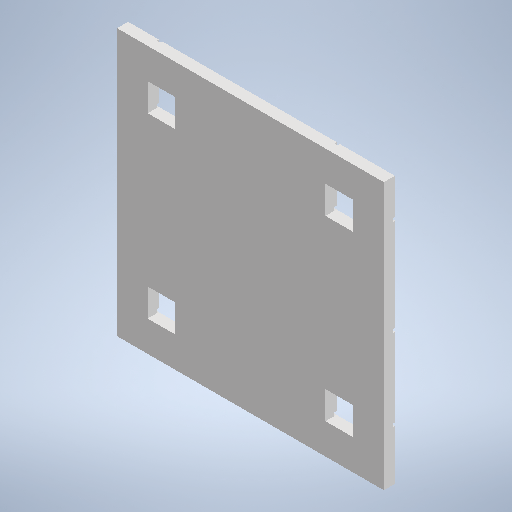
# Autodesk Inventor part: LED Position
Saved by Autodesk Inventor 2025.2 (Build 292293000, 293)
## iProperties
Created: 2025-04-29
Part Number: LED Position
Material: Generic
Document SubType Name: Modeling
Designer: powel
Density: 1 g/cm^3
Appearance: Default
Author: powel
Autodesk Inventor part; units mm, degrees
ref_plane "YZ Plane" through (0, 0, 0) normal (1, 0, 0) x (0, 1, 0)
ref_plane "XZ Plane" through (0, 0, 0) normal (0, 1, 0) x (-1, 0, 0)
ref_plane "XY Plane" through (0, 0, 0) normal (0, 0, 1) x (1, 0, 0)
sketch "Sketch1" plane through (0, 0, 0) normal (0, 0, 1) x (1, 0, 0)
  line L0 (0, 0) -> (48, 0)
  line L1 (48, 0) -> (48, 48)
  line L2 (48, 48) -> (0, 48)
  line L3 (0, 48) -> (0, 0)
  line L4 (10.5, 10.5) -> (5.5, 10.5)
  line L5 (5.5, 10.5) -> (5.5, 5.5)
  line L6 (5.5, 5.5) -> (10.5, 5.5)
  line L7 (10.5, 5.5) -> (10.5, 10.5)
  line L8 (10.5, 10.5) -> (5.5, 5.5) construction
  line L9 (5.5, 10.5) -> (10.5, 5.5) construction
  line L10 (5.5, 42.5) -> (10.5, 42.5)
  line L11 (10.5, 42.5) -> (10.5, 37.5)
  line L12 (10.5, 37.5) -> (5.5, 37.5)
  line L13 (5.5, 37.5) -> (5.5, 42.5)
  line L14 (5.5, 42.5) -> (10.5, 37.5) construction
  line L15 (10.5, 42.5) -> (5.5, 37.5) construction
  line L16 (42.5, 5.5) -> (37.5, 5.5)
  line L17 (37.5, 5.5) -> (37.5, 10.5)
  line L18 (37.5, 10.5) -> (42.5, 10.5)
  line L19 (42.5, 10.5) -> (42.5, 5.5)
  line L20 (42.5, 5.5) -> (37.5, 10.5) construction
  line L21 (37.5, 5.5) -> (42.5, 10.5) construction
  line L22 (42.5, 42.5) -> (37.5, 42.5)
  line L23 (37.5, 42.5) -> (37.5, 37.5)
  line L24 (37.5, 37.5) -> (42.5, 37.5)
  line L25 (42.5, 37.5) -> (42.5, 42.5)
  line L26 (42.5, 42.5) -> (37.5, 37.5) construction
  line L27 (37.5, 42.5) -> (42.5, 37.5) construction
  line L28 (37.5, 5.5) -> (37.5, 6.1)
  line L29 (37.5, 6.1) -> (10.5, 10.5)
  line L30 (37.5, 5.5) -> (10.5, 9.9)
  line L31 (37.5, 37.5) -> (37.5, 38.1)
  line L32 (37.5, 38.1) -> (10.5, 42.5)
  line L33 (37.5, 37.5) -> (10.5, 41.9)
  line L34 (0, 24) -> (0, 23.7)
  line L35 (0, 23.7) -> (48, 23.7)
  line L36 (48, 23.7) -> (48, 24.3)
  line L37 (48, 24.3) -> (0, 24.3)
  line L38 (0, 24.3) -> (0, 23.7)
  line L39 (5.5, 10.5) -> (6.1, 10.5)
  line L40 (6.1, 10.5) -> (6.1, 23.7)
  line L41 (6.1, 23.7) -> (5.5, 23.7)
  line L42 (5.5, 23.7) -> (5.5, 10.5)
  line L43 (10.5, 37.5) -> (9.9, 37.5)
  line L44 (9.9, 37.5) -> (9.9, 24.3)
  line L45 (9.9, 24.3) -> (10.5, 24.3)
  line L46 (10.5, 24.3) -> (10.5, 37.5)
  line L47 (37.5, 10.5) -> (38.1, 10.5)
  line L48 (38.1, 10.5) -> (38.1, 23.7)
  line L49 (38.1, 23.7) -> (37.5, 23.7)
  line L50 (37.5, 23.7) -> (37.5, 10.5)
  line L51 (42.5, 37.5) -> (41.9, 37.5)
  line L52 (41.9, 37.5) -> (41.9, 24.3)
  line L53 (41.9, 24.3) -> (42.5, 24.3)
  line L54 (42.5, 24.3) -> (42.5, 37.5)
  line L55 (10.5, 5.5) -> (9.9, 5.5)
  line L56 (9.9, 5.5) -> (9.9, 0)
  line L57 (9.9, 0) -> (10.5, 0)
  line L58 (10.5, 0) -> (10.5, 5.5)
  line L59 (42.5, 5.5) -> (41.9, 5.5)
  line L60 (41.9, 5.5) -> (41.9, 0)
  line L61 (41.9, 0) -> (42.5, 0)
  line L62 (42.5, 0) -> (42.5, 5.5)
  line L63 (37.5, 42.5) -> (38.1, 42.5)
  line L64 (38.1, 42.5) -> (38.1, 48)
  line L65 (38.1, 48) -> (37.5, 48)
  line L66 (37.5, 48) -> (37.5, 42.5)
  line L67 (5.5, 42.5) -> (6.1, 42.5)
  line L68 (6.1, 42.5) -> (6.1, 48)
  line L69 (6.1, 48) -> (5.5, 48)
  line L70 (5.5, 48) -> (5.5, 42.5)
  line L71 (5.5, 37.5) -> (0, 38.4621)
  line L72 (5.5, 37.5) -> (11.0835, 37.5) construction
  line L73 (5.5, 37.5) -> (5.5, 38.1)
  line L74 (5.5, 38.1) -> (0, 38.9963)
  line L75 (5.5, 5.5) -> (0, 6.4621)
  line L76 (5.5, 5.5) -> (11.0835, 5.5) construction
  line L77 (5.5, 5.5) -> (5.5, 6.1)
  line L78 (5.5, 6.1) -> (0, 6.9963)
  line L79 (42.5, 10.5) -> (48, 9.5379)
  line L80 (42.5, 10.5) -> (48.0835, 10.5) construction
  line L81 (42.5, 10.5) -> (42.5, 9.9)
  line L82 (42.5, 9.9) -> (48, 9.0037)
  line L83 (42.5, 42.5) -> (48, 41.6037)
  line L84 (42.5, 42.5) -> (42.5, 41.9)
  line L85 (42.5, 41.9) -> (48, 41.0037)
  line L86 (6.1, 24.3) -> (9.9, 24.3)
  line L87 (10.5, 24.3) -> (12.4, 24.3)
  arc A0 (12.4, 24.3) -> (8, 24.3) centre (10.2, 24.3124) ccw
  line L88 (5.5, 23.7) -> (3.6, 23.7)
  arc A1 (3.6, 23.7) -> (8, 23.7) centre (5.8, 23.7) ccw
  line L89 (41.9, 24.3) -> (40, 24.3)
  line L90 (42.5, 24.3) -> (44.4, 24.3)
  line L91 (37.5, 23.7) -> (35.6, 23.7)
  arc A2 (35.6, 23.7) -> (40, 23.7) centre (37.8, 23.7) ccw
  arc A3 (44.4, 24.3) -> (40, 24.3) centre (42.2, 24.3124) ccw
  point P0 (8, 24.3)
  point P1 (9.9, 26.4919)
  point P2 (41.9, 26.4919)
  point P3 (10.5, 26.4919)
  point P4 (42.5, 26.4919)
  point P5 (38.1, 21.5205)
  point P6 (37.5, 21.5206)
  point P7 (6.1, 21.5205)
  point P8 (5.5, 21.5206)
  dimension "d33" = 48
  dimension "d34" = 48
  dimension "d38" = 5
  dimension "d39" = 5
  dimension "d40" = 5
  dimension "d41" = 5
  dimension "d45" = 5
  dimension "d46" = 5
  dimension "d47" = 5
  dimension "d48" = 5
  dimension "d49" = 32
  dimension "d50" = 32
  dimension "d51" = 32
  dimension "d52" = 32
  dimension "d53" = 0.6
  dimension "d54" = 0.6
  dimension "d55" = 0.3
  dimension "d56" = 0.6
  dimension "d57" = 0.6
  dimension "d58" = 0.6
  dimension "d59" = 0.6
  dimension "d60" = 0.6
  dimension "d61" = 0.6
  dimension "d62" = 0.6
  dimension "d63" = 0.6
  dimension "d64" = 0.6
  dimension "d65" = 170.078
  dimension "d66" = 0.6
  dimension "d67" = 170.078
  dimension "d68" = 0.6
  dimension "d69" = 9.922
  dimension "d70" = 0.6
  dimension "d71" = 0.6
  dimension "d72" = 1.9
  dimension "d73" = 1.9
  dimension "d74" = 1.9
  dimension "d75" = 1.9
  dimension "d76" = 1.9
  dimension "d77" = 1.9
  constraints: 184 end point, 34 point on line, 33 parallel, 17 horizontal, 14 perpendicular, 8 point on circle, 4 centre point, 3 equal length, 2 midpoint, 1 collinear
  measures "d33" distance of L2.end L1.end
  measures "d34" distance of L1.end L0.end
  measures "d38" distance of L6.end L5.end
  measures "d39" distance of L5.end L4.end
  measures "d40" distance of L11.end L12.end
  measures "d41" distance of L10.end L11.end
  measures "d45" distance of L17.end L18.end
  measures "d46" distance of L16.end L17.end
  measures "d47" distance of L24.end L23.end
  measures "d48" distance of L23.end L22.end
  measures "d49" distance of L24.end L11.end
  measures "d50" distance of L16.end L23.end
  measures "d51" distance of L4.end L17.end
  measures "d52" distance of L10.end L4.start
  measures "d53" distance of L16.end L28.end
  measures "d54" distance of L23.end L31.end
  measures "d55" distance of L34.start L34.end
  measures "d56" distance of L36.end L35.end
  measures "d57" distance of L41.end L40.end
  measures "d58" distance of L45.end L44.end
  measures "d59" distance of L49.end L48.end
  measures "d60" distance of L53.end L52.end
  measures "d61" distance of L57.end L56.end
  measures "d62" distance of L61.end L60.end
  measures "d63" distance of L65.end L64.end
  measures "d64" distance of L69.end L68.end
  measures "d65" angle of L72 L71
  measures "d66" distance of L12.end L73.end
  measures "d67" angle of L76 L75
  measures "d68" distance of L5.end L77.end
  measures "d69" angle of L79 L80
  measures "d70" distance of L18.end L81.end
  measures "d71" distance of L22.start L84.end
  measures "d72" distance of L44.end A0.end
  measures "d73" distance of L45.end L87.end
  measures "d74" distance of L41.end L88.end
  measures "d75" distance of L52.end L89.end
  measures "d76" distance of L53.end L90.end
  measures "d77" distance of L49.end L91.end
extrude "Extrusion1" add sketch "Sketch1" against normal blind 0.4 contours L3 L75 L6 L56 L0 | L58 L7 L30 L16 L60 L0 | L3 L35 A1 L42 L5 L78 | L62 L19 L82 L1 L0 | L4 L40 A1 L35 A2 L50 L17 L29 | L3 L71 L12 L44 A0 L37 | L79 L18 L48 A2 L35 L1 | L3 L2 L70 L13 L74 | L37 A3 L54 L25 L85 L1 | L11 L33 L24 L52 A3 L37 A0 L46 | L2 L66 L23 L32 L10 L68 | L83 L22 L64 L2 L1
extrude "Extrusion2" add sketch "Sketch1" along normal blind 1.6 contours L3 L75 L6 L56 L0 | L56 L6 L58 L0 | L3 L78 L5 L75 | L58 L7 L30 L16 L60 L0 | L3 L35 A1 L42 L5 L78 | L60 L16 L62 L0 | L3 L37 L1 L35 | L62 L19 L82 L1 L0 | L7 L29 L17 L30 | L35 L42 A1 | L42 A1 L40 L4 | L4 L40 A1 L35 A2 L50 L17 L29 | L3 L71 L12 L44 A0 L37 | L35 L40 A1 L42 | L82 L19 L79 L1 | L3 L74 L13 L71 | L35 A1 L40 | L79 L18 L48 A2 L35 L1 | L50 A2 L48 L18 | L3 L2 L70 L13 L74 | A0 L44 L37 | A2 L35 L50 | L50 L35 L48 A2 | L12 L46 A0 L44 | L44 A0 L46 L37 | L37 A3 L54 L25 L85 L1 | A2 L48 L35 | L2 L68 L10 L70 | L11 L33 L24 L52 A3 L37 A0 L46 | L46 A0 L37 | L85 L25 L83 L1 | L37 L54 A3 | L2 L66 L23 L32 L10 L68 | L11 L32 L23 L33 | L83 L22 L64 L2 L1 | L37 L52 A3 L54 | A3 L52 L24 L54 | L2 L64 L22 L66 | A3 L52 L37
body "Solid1"
